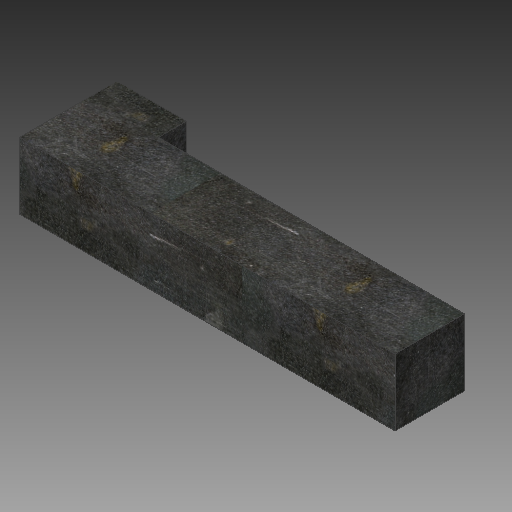
# Autodesk Inventor part: ventilador_tangencial_referencia
Saved by Autodesk Inventor 2018 (Build 220112000, 112)
## iProperties
Created: 2018-05-16
Part Number: ventilador_tangencial_referencia
Material: Aço
Document SubType Name: Modeling
Designer: Usuario
Density: 7.85 g/cm^3
Appearance: Placa
Author: Usuario
Autodesk Inventor part; units mm, degrees
ref_plane "YZ Plane" through (0, 0, 0) normal (1, 0, 0) x (0, 1, 0)
ref_plane "XZ Plane" through (0, 0, 0) normal (0, 1, 0) x (-1, 0, 0)
ref_plane "XY Plane" through (0, 0, 0) normal (0, 0, 1) x (1, 0, 0)
sketch "Esboço1" plane through (0, 0, 0) normal (0, 0, 1) x (1, 0, 0)
  line L0 (-110, 24) -> (110, 24)
  line L1 (110, 24) -> (110, -24)
  line L2 (110, -24) -> (-110, -24)
  line L3 (-110, -24) -> (-110, 24)
  line L4 (-110, 24) -> (110, -24) construction
  line L5 (110, 24) -> (-110, -24) construction
  point P0 (0, 0)
  dimension "d0" = 220
  dimension "d1" = 48
  constraints: 12 end point, 2 midpoint, 2 parallel, 1 horizontal, 1 perpendicular
  measures "d0" distance of L1.end L2.end
  measures "d1" distance of L0.end L1.end
extrude "Extrusão1" add sketch "Esboço1" along normal blind 50
sketch "Esboço2" plane through (-110, -24, 0) normal (-1, 0, 0) x (0, 0, 1)
  line L0 (50, 48) -> (50, 0) construction
  line L1 (0, 48) -> (50, 48) construction
  line L2 (50, 48) -> (50, 0) construction
  line L3 (50, 0) -> (0, 0) construction
  line L4 (0, 0) -> (0, 48) construction
  line L5 (0, 48) -> (50, 0) construction
  line L6 (50, 48) -> (0, 0) construction
  line L7 (0, 48) -> (-20, 48) construction
  line L8 (-20, 48) -> (-20, 0) construction
  line L9 (-20, 0) -> (0, 0) construction
  line L10 (-20, 24) -> (15, 24) construction
  line L11 (50, 48) -> (-20, 48)
  line L12 (-20, 48) -> (-20, 0)
  line L13 (-20, 0) -> (50, 0)
  line L14 (50, 0) -> (50, 48)
  line L15 (50, 48) -> (-20, 0) construction
  line L16 (-20, 48) -> (50, 0) construction
  point P0 (0, 24)
  point P1 (25, 24)
  dimension "d4" = 20
  dimension "d5" = 35
  constraints: 32 end point, 5 midpoint, 4 horizontal, 4 parallel, 4 perpendicular
  measures "d4" distance of L1.start L7.end
  measures "d5" distance of L10.start L10.end
extrude "Extrusão2" add sketch "Esboço2" along normal blind 50
